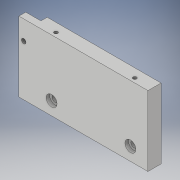
# Autodesk Inventor part: right side
Saved by Autodesk Inventor 2017 (Build 210142000, 142)
## iProperties
Created: 2016-07-21
Part Number: right side
Material: Generic
Document SubType Name: Modeling
Designer: Darien Morrow
Density: 1 g/cm^3
Appearance: Default
Author: Darien Morrow
Autodesk Inventor part; units mm, degrees
ref_plane "YZ Plane" through (0, 0, 0) normal (1, 0, 0) x (0, 1, 0)
ref_plane "XZ Plane" through (0, 0, 0) normal (0, 1, 0) x (-1, 0, 0)
ref_plane "XY Plane" through (0, 0, 0) normal (0, 0, 1) x (1, 0, 0)
sketch "Sketch1" plane through (0, 0, 0) normal (0, 0, 1) x (1, 0, 0)
  line L0 (-41.275, -25.4) -> (41.275, -25.4)
  line L1 (41.275, -25.4) -> (41.275, 25.4)
  line L2 (41.275, 25.4) -> (-41.275, 25.4)
  line L3 (-41.275, 25.4) -> (-41.275, -25.4)
  line L4 (-41.275, -25.4) -> (41.275, 25.4) construction
  line L5 (41.275, -25.4) -> (-41.275, 25.4) construction
  point P0 (0, 0)
  dimension "d0" = 82.55
  dimension "d1" = 50.8
  constraints: 12 end point, 2 midpoint, 2 parallel, 1 horizontal, 1 perpendicular
  measures "d0" distance of L2.end L1.end
  measures "d1" distance between parallel lines of L0 L2
extrude "Extrusion1" add sketch "Sketch1" along normal blind 9.525
sketch "Sketch2" plane through (0, 0, 9.525) normal (0, 0, 1) x (1, 0, 0)
  line L0 (-28.575, -15.875) -> (28.575, -15.875)
  line L1 (-41.275, 25.4) -> (-41.275, -25.4) projected
  line L2 (-41.275, -25.4) -> (41.275, -25.4) projected
  point P0 (0, 0)
  dimension "d4" = 57.15
  dimension "d5" = 12.7
  dimension "d6" = 9.525
  constraints: 2 coincident, 2 end point, 1 horizontal
  measures "d4" distance of L0.start L0.end
  measures "d5" distance from line of L1 L0.start
  measures "d6" distance between parallel lines of L0 L2
hole "Hole1" at (-28.575, -15.875, 9.525) at (28.575, -15.875, 9.525) direction (0, 0, -1) diameter 4.4958 depth 25.4 tip angle 118 counterbore diameter 7.9502 counterbore depth 2.54 clearance for "Socket Head Cap Screw" size "#8" standard "Ansi Unified Screw Threads"
sketch "Sketch3" plane through (0, 0, 9.525) normal (0, 0, 1) x (1, 0, 0)
  line L0 (-41.275, 25.4) -> (-41.275, -25.4) projected
  line L1 (-41.275, -25.4) -> (-41.275, 25.4)
  line L2 (-41.275, 25.4) -> (-52.275, 25.4)
  line L3 (-52.275, 25.4) -> (-52.275, -25.4)
  line L4 (-52.275, -25.4) -> (-41.275, -25.4)
  point P0 (0, 0)
  dimension "d14" = 11
  constraints: 8 end point, 3 equal length, 1 perpendicular
  measures "d14" distance of L2.end L0.start
extrude "Extrusion2" add sketch "Sketch3" against normal blind 4.953
sketch "Sketch4" plane through (0, 0, 4.572) normal (0, 0, -1) x (-1, 0, 0)
  line L0 (52.275, 25.4) -> (41.275, 25.4) projected
  line L1 (52.275, -25.4) -> (52.275, 25.4) projected
  point P0 (0, 0)
  point P1 (48.775, 11.43)
  dimension "d17" = 13.97
  dimension "d18" = 3.5
  measures "d17" distance from line of point (48.775, 11.43) L0
  measures "d18" distance from line of L1 point (48.775, 11.43)
hole "Hole2" at (-48.775, 11.43, 4.572) direction (0, 0, 1) diameter 3.302 depth 12.2936 tip angle 118 thread size "8-32 UNC" class "2B" standard "ANSI Unified Screw Threads"
sketch "Sketch5" plane through (-41.275, 25.4, 0) normal (0, 1, 0) x (1, 0, 0)
  line L0 (69.85, -6.35) -> (12.7, -6.35)
  line L1 (0, 0) -> (0, -4.572) projected
  line L2 (82.55, -9.525) -> (-11, -9.525) projected
  point P0 (41.275, 0)
  dimension "d26" = 57.15
  dimension "d27" = 12.7
  dimension "d28" = 3.175
  constraints: 2 coincident, 2 end point, 1 horizontal
  measures "d26" distance of L0.start L0.end
  measures "d27" distance from line of L0.end L1
  measures "d28" distance between parallel lines of L0 L2
hole "Hole3" at (-28.575, 25.4, 6.35) at (28.575, 25.4, 6.35) direction (0, -1, 0) diameter 2.6416 depth 10.9728 tip angle 118 thread size "6-32 UNC" class "2B" standard "ANSI Unified Screw Threads"
body "Solid1"
